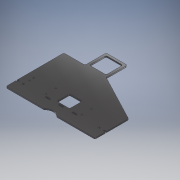
# Autodesk Inventor part: EXTERNAL SIDE PLATE
Saved by Autodesk Inventor 2018 (Build 220112000, 112)
## iProperties
Created: 2018-10-15
Part Number: EXTERNAL SIDE PLATE
Material: Acero, carbono
Document SubType Name: Modeling
Designer: Toshiba
Density: 7.85 g/cm^3
Appearance: Mecanizado 02
Author: Toshiba
Autodesk Inventor part; units mm, degrees
ref_plane "YZ Plane" through (0, 0, 0) normal (1, 0, 0) x (0, 1, 0)
ref_plane "XZ Plane" through (0, 0, 0) normal (0, 1, 0) x (-1, 0, 0)
ref_plane "XY Plane" through (0, 0, 0) normal (0, 0, 1) x (1, 0, 0)
sketch "Boceto1" plane through (0, 0, 0) normal (0, 0, 1) x (1, 0, 0)
  line L0 (200, -155) -> (-200, -155)
  line L1 (-200, -155) -> (-200, 105)
  line L2 (-200, 105) -> (-105, 105)
  line L3 (-105, 105) -> (-105, 200)
  line L4 (-105, 200) -> (-10, 200)
  line L5 (-10, 200) -> (-10, 105)
  line L6 (200, -155) -> (200, -5)
  line L7 (200, -5) -> (-10, 105)
  line L8 (-27.6071, -98.5) -> (29.3929, -98.5)
  line L9 (29.3929, -98.5) -> (29.3929, -41.5)
  line L10 (29.3929, -41.5) -> (-27.6071, -41.5)
  line L11 (-27.6071, -41.5) -> (-27.6071, -98.5)
  line L12 (-27.6071, -98.5) -> (29.3929, -41.5) construction
  line L13 (29.3929, -98.5) -> (-27.6071, -41.5) construction
  line L14 (-20, 115) -> (-95, 115)
  line L15 (-95, 115) -> (-95, 190)
  line L16 (-95, 190) -> (-20, 190)
  line L17 (-20, 190) -> (-20, 115)
  line L18 (-20, 115) -> (-95, 190) construction
  line L19 (-95, 115) -> (-20, 190) construction
  point P0 (0.8929, -70)
  point P1 (-57.5, 152.5)
  dimension "d2" = 260
  dimension "d3" = 95
  dimension "d4" = 95
  dimension "d5" = 150
  dimension "d6" = 400
  dimension "d7" = 57
  dimension "d8" = 57
  dimension "d10" = 75
  dimension "d11" = 75
  constraints: 40 end point, 5 horizontal, 4 midpoint, 4 parallel, 4 perpendicular, 4 vertical
  measures "d2" distance of L0.end L1.end
  measures "d3" distance of L1.end L2.end
  measures "d4" distance of L3.end L4.end
  measures "d5" distance of L0.start L6.end
  measures "d6" distance of L0.start L0.end
  measures "d7" distance of L10.end L9.end
  measures "d8" distance of L9.end L8.end
  measures "d10" distance of L15.end L16.end
  measures "d11" distance of L14.end L15.end
extrude "Extrusión1" add sketch "Boceto1" along normal blind 6
fillet "Empalme1" radius 6 16 edges at (-10, 105, 3) (-10, 200, 3) (200, -5, 3) (200, -155, 3) (-200, -155, 3) (-200, 105, 3) (-105, 105, 3) (-105, 200, 3) (-95, 190, 3) (-20, 190, 3) (-20, 115, 3) (-95, 115, 3) (-27.6071, -41.5, 3) (29.3929, -41.5, 3) (29.3929, -98.5, 3) (-27.6071, -98.5, 3)
sketch "Boceto2" plane through (0, 0, 6) normal (0, 0, 1) x (1, 0, 0)
  line L0 (10, -110) -> (-10, -110)
  line L1 (-10, -110) -> (-10, -104)
  line L2 (-10, -104) -> (10, -104)
  line L3 (10, -104) -> (10, -110)
  line L4 (10, -110) -> (-10, -104) construction
  line L5 (-10, -110) -> (10, -104) construction
  line L6 (-194, -155) -> (194, -155) projected
  line L7 (-50, -110) -> (-70, -110)
  line L8 (-70, -110) -> (-70, -104)
  line L9 (-70, -104) -> (-50, -104)
  line L10 (-50, -104) -> (-50, -110)
  line L11 (-50, -110) -> (-70, -104) construction
  line L12 (-70, -110) -> (-50, -104) construction
  line L13 (70, -110) -> (50, -110)
  line L14 (50, -110) -> (50, -104)
  line L15 (50, -104) -> (70, -104)
  line L16 (70, -104) -> (70, -110)
  line L17 (70, -110) -> (50, -104) construction
  line L18 (50, -110) -> (70, -104) construction
  circle A0 centre (-170, -107) radius 4
  line L19 (-190, -110) -> (-210, -110)
  line L20 (-210, -110) -> (-210, -104)
  line L21 (-210, -104) -> (-190, -104)
  line L22 (-190, -104) -> (-190, -110)
  line L23 (-200, -149) -> (-200, 99) projected
  line L24 (-190, -110) -> (-210, -104) construction
  line L25 (-210, -110) -> (-190, -104) construction
  circle A1 centre (-80, -95) radius 3
  circle A2 centre (-80, -51) radius 3
  circle A3 centre (-170, -80) radius 3
  circle A4 centre (-170, -60) radius 3
  line L26 (0, 0) -> (0, -107)
  circle A5 centre (170, -107) radius 4
  line L27 (190, -110) -> (210, -110)
  line L28 (210, -110) -> (210, -104)
  line L29 (210, -104) -> (190, -104)
  line L30 (190, -104) -> (190, -110)
  circle A6 centre (80, -95) radius 3
  circle A7 centre (80, -51) radius 3
  line L31 (194, -155) -> (-194, -155) projected
  arc A8 (29.2, -155) -> (-29.2, -155) centre (0, -182.3379) ccw
  line L32 (-29.2, -155) -> (29.2, -155)
  point P0 (-60, -107)
  point P1 (60, -107)
  point P2 (-200, -107)
  dimension "d15" = 20
  dimension "d16" = 6
  dimension "d17" = 48
  dimension "d18" = 20
  dimension "d19" = 60
  dimension "d20" = 20
  dimension "d21" = 60
  dimension "d22" = 8
  dimension "d23" = 20
  dimension "d24" = 6
  dimension "d25" = 110
  dimension "d26" = 6
  dimension "d27" = 20
  dimension "d28" = 12
  dimension "d29" = 6
  dimension "d30" = 44
  dimension "d31" = 6
  dimension "d32" = 6
  dimension "d33" = 40
  dimension "d36" = 6
  dimension "d37" = 6
  constraints: 60 end point, 9 centre point, 8 midpoint, 8 parallel, 7 symmetric about line, 5 perpendicular, 4 horizontal, 3 point on line, 2 point on circle, 1 collinear, 3 other
  measures "d15" distance of L1.end L2.end
  measures "d16" distance of L0.end L1.end
  measures "d17" distance from line of L6 L26.end
  measures "d18" distance of L8.end L9.end
  measures "d19" distance of point (-60, -107) L26.end
  measures "d20" distance of L14.end L15.end
  measures "d21" distance of point (60, -107) L26.end
  measures "d22" diameter of A0
  measures "d23" distance of L20.end L21.end
  measures "d24" distance of L19.end L20.end
  measures "d25" distance of point (-60, -107) A0.centre
  measures "d26" diameter of A1
  measures "d27" horizontal distance of A1.centre point (-60, -107)
  measures "d28" vertical distance of point (-60, -107) A1.centre
  measures "d29" diameter of A2
  measures "d30" distance of A1.centre A2.centre
  measures "d31" diameter of A3
  measures "d32" diameter of A4
  measures "d33" radius of A8
  measures "d36" distance of L9.end L7.start
  measures "d37" distance of L15.end L13.start
extrude "Extrusión2" cut sketch "Boceto2" against normal through all
